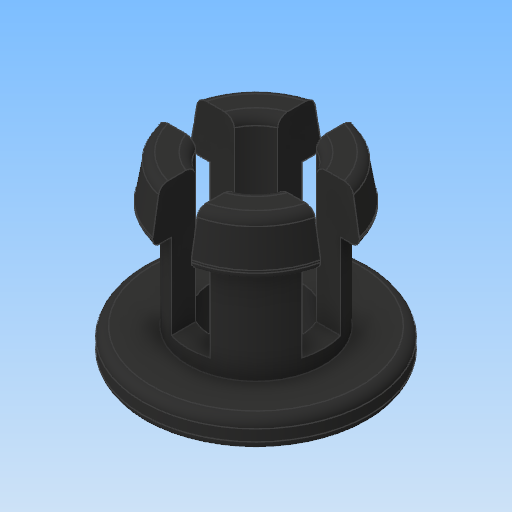
# Autodesk Inventor part: NF-Crazy   фитинг
Saved by Autodesk Inventor 2017 (Build 210142000, 142)
## iProperties
Part Number: NF-Crazy   фитинг
Material: Типовые
Document SubType Name: Modeling
Designer: chucha
Density: 1 g/cm^3
Appearance: Резина — черная
Mass: 0.16684 g
Surface Area: 3.89817 cm^2
Volume: 0.16684 cm^3
Author: chucha
Autodesk Inventor part; units mm, degrees
ref_plane "YZ Plane" through (0, 0, 0) normal (1, 0, 0) x (0, 1, 0)
ref_plane "XZ Plane" through (0, 0, 0) normal (0, 1, 0) x (-1, 0, 0)
ref_plane "XY Plane" through (0, 0, 0) normal (0, 0, 1) x (1, 0, 0)
sketch "Эскиз1" plane through (0, 0, 0) normal (0, 0, 1) x (1, 0, 0)
  line L0 (0, 0) -> (0, 11.7004) construction
  line L1 (0, 0) -> (-23.4572, 0) construction
  line L2 (0, 0) -> (-5, 0)
  line L3 (-5, 0) -> (-5, 1.3)
  line L4 (-5, 1.3) -> (-3, 1.3)
  line L5 (-3, 1.3) -> (-3, 5.7)
  line L6 (-3, 5.7) -> (-3.8, 5.7)
  line L7 (-3.8, 5.7) -> (-3.8, 6.1)
  line L8 (-3.8, 6.1) -> (-3.5, 7.94)
  line L9 (-3.5, 7.94) -> (-2, 7.94)
  line L10 (-2, 7.94) -> (-2, 0)
  dimension "d0" = 5
  dimension "d1" = 1.3
  dimension "d2" = 3
  dimension "d3" = 4.4
  dimension "d4" = 2
  dimension "d5" = 7.94
  dimension "d6" = 3.5
  dimension "d8" = 3.8
  dimension "d9" = 0.4
  constraints: 22 end point, 6 perpendicular, 2 point on line, 2 vertical, 1 parallel
  measures "d0" distance of L0.start L2.end
  measures "d1" distance of L2.end L3.end
  measures "d2" distance from line of L0 L4.end
  measures "d3" distance of L4.end L5.end
  measures "d4" distance between parallel lines of L0 L10
  measures "d5" distance between parallel lines of L1 L9
  measures "d6" distance from line of L0 L8.end
  measures "d8" distance between parallel lines of L0 L7
  measures "d9" distance of L6.end L7.end
revolve "Вращение1" add sketch "Эскиз1" angle 360 about axis through (0, 0, 0) along (0, 1, 0)
fillet "Сопряжение1" radius 0.4 2 edges at (5, 1.3, 0) (5, 0, 0)
fillet "Сопряжение2" radius 0.3 1 edges at (3.8, 5.7, 0)
fillet "Сопряжение3" radius 0.4 2 edges at (3.5, 7.94, 0) (2, 7.94, 0)
sketch "Эскиз2" plane through (0, 7.94, 0) normal (0, 1, 0) x (1, 0, 0)
  line L0 (-10.37, -0.85) -> (10.2464, -0.85)
  line L1 (10.2464, -0.85) -> (10.2464, 0.85)
  line L2 (10.2464, 0.85) -> (-10.37, 0.85)
  line L3 (-10.37, 0.85) -> (-10.37, -0.85)
  line L4 (-0.85, -12.4719) -> (0.85, -12.4719)
  line L5 (0.85, -12.4719) -> (0.85, 12.1626)
  line L6 (0.85, 12.1626) -> (-0.85, 12.1626)
  line L7 (-0.85, 12.1626) -> (-0.85, -12.4719)
  line L8 (0, 0) -> (-10.37, 0) construction
  line L9 (0, 0) -> (0, -12.4719) construction
  dimension "d14" = 1.7
  dimension "d15" = 1.7
  constraints: 20 end point, 4 parallel, 3 perpendicular, 2 horizontal, 2 midpoint, 2 other
  measures "d14" distance between parallel lines of L0 L2
  measures "d15" distance between parallel lines of L5 L7
extrude "Выдавливание1" cut sketch "Эскиз2" against normal blind 6
